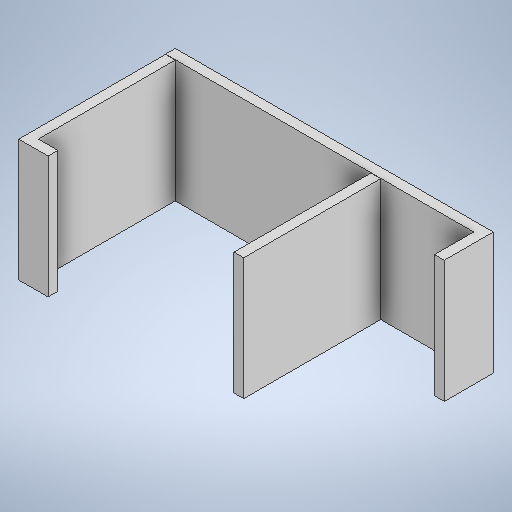
# Autodesk Inventor part: PwrStrpHLDR
Saved by Autodesk Inventor 2025.1 (Build 291241000, 241)
## iProperties
Created: 2024-11-24
Part Number: PwrStrpHLDR
Material: Generic
Document SubType Name: Modeling
Designer: shubh
Density: 1 g/cm^3
Appearance: Default
Author: shubh
Autodesk Inventor part; units mm, degrees
ref_plane "YZ Plane" through (0, 0, 0) normal (1, 0, 0) x (0, 1, 0)
ref_plane "XZ Plane" through (0, 0, 0) normal (0, 1, 0) x (-1, 0, 0)
ref_plane "XY Plane" through (0, 0, 0) normal (0, 0, 1) x (1, 0, 0)
sketch "Sketch3" plane through (0, 0, 0) normal (0, 0, 1) x (1, 0, 0)
  line L0 (32.5, -12.5) -> (-32.5, -12.5)
  line L1 (-32.5, -12.5) -> (-32.5, 12.5)
  line L2 (-32.5, 12.5) -> (32.5, 12.5)
  line L3 (32.5, 12.5) -> (32.5, -12.5)
  line L4 (32.5, -12.5) -> (-32.5, 12.5) construction
  line L5 (-32.5, -12.5) -> (32.5, 12.5) construction
  point P0 (0, 0)
  dimension "d4" = 65
  dimension "d5" = 25
  constraints: 12 end point, 2 midpoint, 2 parallel, 1 horizontal, 1 perpendicular
  measures "d4" distance of L1.end L2.end
  measures "d5" distance of L0.end L1.end
extrude "Extrusion2" add sketch "Sketch3" along normal blind 2
sketch "Sketch4" plane through (0, 0, 2) normal (0, 0, 1) x (1, 0, 0)
  line L0 (-32.5, -12.5) -> (32.5, -12.5) projected
  line L1 (-32.5, 12.4423) -> (-30.5, 12.4423)
  line L2 (-30.5, 12.4423) -> (-30.5, -12.5)
  line L3 (-30.5, -12.5) -> (-32.5, -12.5)
  line L4 (-32.5, -12.5) -> (-32.5, 12.4423)
  line L5 (9.5, 12.4423) -> (11.5, 12.4423)
  line L6 (11.5, 12.4423) -> (11.5, -12.5)
  line L7 (11.5, -12.5) -> (9.5, -12.5)
  line L8 (9.5, -12.5) -> (9.5, 12.4423)
  line L9 (30.5, 12.4423) -> (32.5, 12.4423)
  line L10 (32.5, 12.4423) -> (32.5, -12.5)
  line L11 (32.5, -12.5) -> (30.5, -12.5)
  line L12 (30.5, -12.5) -> (30.5, 12.4423)
  line L13 (32.5, -12.5) -> (32.5, 12.5) projected
  line L14 (-32.5, 12.5) -> (-32.5, -12.5) projected
  point P0 (0, 0)
  point P1 (11.5, -12.5)
  dimension "d8" = 2
  dimension "d9" = 2
  dimension "d10" = 2
  dimension "d11" = 19
  constraints: 24 end point, 6 parallel, 3 collinear, 3 horizontal, 3 perpendicular, 3 point on line
  measures "d8" distance of L2.end L3.end
  measures "d9" distance of L6.end L7.end
  measures "d10" distance of L10.end L11.end
  measures "d11" distance between parallel lines of L12 L6
extrude "Extrusion3" add sketch "Sketch4" along normal blind 28 contours L4 L1 L2 L0 | L8 L5 L6 L0
sketch "Sketch5" plane through (0, 0, 2) normal (0, 0, 1) x (1, 0, 0)
  line L0 (32.5, 12.5) -> (-32.5, 12.5) projected
  line L1 (11.5, -12.5) -> (32.5, -12.5) projected
  line L2 (32.5, 12.5) -> (30.5, 12.5)
  line L3 (30.5, 12.5) -> (30.5, -12.5)
  line L4 (30.5, -12.5) -> (32.5, -12.5)
  line L5 (32.5, -12.5) -> (32.5, 12.5)
  line L6 (32.5, -12.5) -> (32.5, 12.5) projected
  point P0 (0, 0)
  dimension "d14" = 2
  constraints: 8 end point, 2 parallel, 1 collinear, 1 horizontal, 1 perpendicular, 1 point on line
  measures "d14" distance of L4.end L3.end
extrude "Extrusion4" add sketch "Sketch5" along normal blind 8
sketch "Sketch6" plane through (-32.5, -12.5, 0) normal (-1, 0, 0) x (0, 0, 1)
  point P0 (0, 12.5)
sketch "Sketch7" plane through (-32.5, -12.5, 0) normal (-1, 0, 0) x (0, 0, 1)
  line L0 (2, 24.9423) -> (30, 24.9423) projected
  line L1 (30, 24.9423) -> (32, 24.9423)
  line L2 (32, 24.9423) -> (32, 0)
  line L3 (32, 0) -> (30, 0)
  line L4 (30, 0) -> (30, 24.9423)
  point P0 (0, 12.5)
  dimension "d17" = 2
  constraints: 8 end point, 2 parallel, 1 horizontal, 1 perpendicular, 1 point on line
  measures "d17" distance of L2.end L3.end
extrude "Extrusion5" add sketch "Sketch7" against normal blind 6
body "Solid2"
